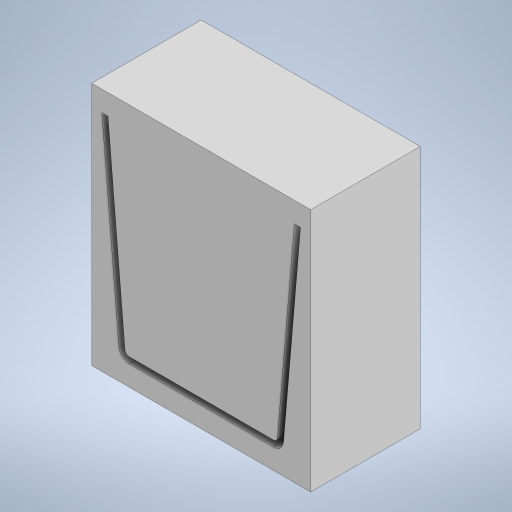
# Autodesk Inventor part: molde_vaso
Saved by Autodesk Inventor 2023.2 (Build 272271030, 271C)
## iProperties
Created: 2023-07-24
Part Number: molde_vaso
Material: Generic
Document SubType Name: Modeling
Designer: Cris Pat
Density: 1 g/cm^3
Appearance: Default
Author: Cris Pat
Autodesk Inventor part; units mm, degrees
ref_plane "YZ Plane" through (0, 0, 0) normal (1, 0, 0) x (0, 1, 0)
ref_plane "XZ Plane" through (0, 0, 0) normal (0, 1, 0) x (-1, 0, 0)
ref_plane "XY Plane" through (0, 0, 0) normal (0, 0, 1) x (1, 0, 0)
sketch "Sketch1" plane through (0, 0, 0) normal (0, 1, 0) x (-1, 0, 0)
  circle A0 centre (0, 0) radius 40
  dimension "d0" = 80
  constraints: 1 centre point, 1 coincident
  measures "d0" diameter of A0
extrude "Extrusion1" add sketch "Sketch1" along normal blind 100 draft 5
fillet "Fillet1" radius 5 1 edges at (40, 0, 0)
shell "Shell1" thickness 3 removed faces 1 at (0.3523, 100, 10.6656)
sketch "Sketch2" plane through (0, 0, 0) normal (0, 1, 0) x (-1, 0, 0)
  line L0 (53.7489, -53.7489) -> (-53.7489, -53.7489)
  line L1 (-53.7489, -53.7489) -> (-53.7489, 53.7489)
  line L2 (-53.7489, 53.7489) -> (53.7489, 53.7489)
  line L3 (53.7489, 53.7489) -> (53.7489, -53.7489)
  circle A0 centre (0, 0) radius 48.7489 construction
  circle A1 centre (0, 0) radius 53.7489 construction
  dimension "d5" = 5
  constraints: 8 end point, 4 tangent, 2 parallel, 1 centre point, 1 horizontal, 1 perpendicular
  measures "d5" radial gap between concentric circles of A0 A1
extrude "Extrusion2" add sketch "Sketch2" along normal blind 110 and the other way blind 10 separate body
combine bodies "Combine1" operation type subtract main body 2 bodies to subtract 1
split body "Split1" result two bodies by plane through (0, 0, 0) normal (0, 0, 1) bodies 2 first body at (44.8681, 52.2385, 4.2844)
body "Solid3"
body "Solid4"
